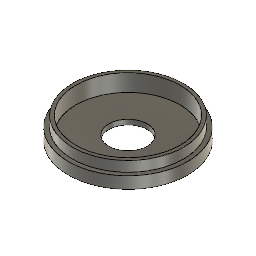
build-button-lid (Autodesk Fusion 360 design; units mm, degrees)
Autodesk Fusion 360 part; units mm, degrees
ref_plane "WorkPlane5" through (0, 0, 0) normal (0, 0, 1) x (1, 0, 0)
sketch "Sketch6" plane through (0, 0, 0) normal (0, 0, 1) x (1, 0, 0)
  circle A0 centre (0, 0) radius 35
  circle A1 centre (0, 0) radius 11.25
  circle A2 centre (0, 0) radius 32.5
  circle A3 centre (0, 0) radius 30.5
  circle A4 centre (0, 0) radius 33
  dimension "d64" = 22.5
  dimension "d73" = 70
  dimension "d75" = 66
  dimension "d77" = 0.5
  dimension "d78" = 2
  measures "d64" diameter of A1
  measures "d73" diameter of A0
  measures "d75" diameter of A4
  measures "d77" distance of A2 A4
  measures "d78" distance of A2 A3
extrude "Extrude15" add sketch "Sketch6" against normal blind 3 contours A0 | A2 | A3 | A4
extrude "Extrude16" add sketch "Sketch6" against normal blind 7 contours A0 | A2 | A4
extrude "Extrude17" add sketch "Sketch6" against normal blind 13 contours A2
move_body "Move1" bodies 1 to x (1, 0, 0) y (0, 1, 0) z (0, 0, 1) at (0, 0, -43)
move_body "Move2" bodies 1 to x (1, 0, 0) y (0, 1, 0) z (0, 0, 1) at (0, 0, 55)
move_body "Move3" bodies 1 to x (-1, 0, 0) y (0, 1, 0) z (0, 0, -1) at (-57.5753, 12.4946, -1.9302)
named bodies: "lid"
